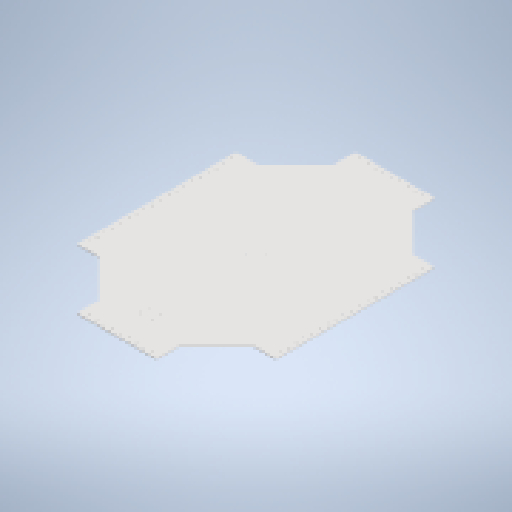
# Autodesk Inventor part: Baseplate V2.1
Saved by Autodesk Inventor 2023 (Build 270158000, 158)
## iProperties
Created: 2023-01-16
Part Number: Baseplate V2.1
Material: Generic
Document SubType Name: Modeling
Designer: Gabriel - T3 CAD
Density: 1 g/cm^3
Appearance: Default
Author: Gabriel - T3 CAD
Autodesk Inventor part; units mm, degrees
ref_plane "YZ Plane" through (0, 0, 0) normal (1, 0, 0) x (0, 1, 0)
ref_plane "XZ Plane" through (0, 0, 0) normal (0, 1, 0) x (-1, 0, 0)
ref_plane "XY Plane" through (0, 0, 0) normal (0, 0, 1) x (1, 0, 0)
sketch "Sketch1" plane through (0, 0, 0) normal (0, 1, 0) x (-1, 0, 0)
  line L0 (0, 0) -> (635, 0)
  line L1 (635, 0) -> (635, 889)
  line L2 (635, 889) -> (0, 889)
  line L3 (0, 889) -> (0, 0)
  line L4 (0, 0) -> (69.85, 0)
  line L5 (69.85, 0) -> (69.85, 190.5)
  line L6 (69.85, 190.5) -> (0, 190.5)
  line L7 (0, 190.5) -> (0, 0)
  line L8 (0, 0) -> (190.5, 0)
  line L9 (190.5, 0) -> (190.5, 69.85)
  line L10 (190.5, 69.85) -> (0, 69.85)
  line L11 (0, 69.85) -> (0, 0)
  line L12 (190.5, 69.85) -> (69.85, 190.5)
  line L13 (317.5, 889) -> (317.5, 0)
  line L14 (0, 444.5) -> (635, 444.5)
  line L15 (565.15, 0) -> (565.15, 190.5)
  line L16 (565.15, 190.5) -> (635, 190.5)
  line L17 (444.5, 0) -> (444.5, 69.85)
  line L18 (444.5, 69.85) -> (635, 69.85)
  line L19 (444.5, 69.85) -> (565.15, 190.5)
  line L20 (69.85, 889) -> (69.85, 698.5)
  line L21 (69.85, 698.5) -> (0, 698.5)
  line L22 (190.5, 889) -> (190.5, 819.15)
  line L23 (190.5, 819.15) -> (0, 819.15)
  line L24 (190.5, 819.15) -> (69.85, 698.5)
  line L25 (565.15, 889) -> (565.15, 698.5)
  line L26 (565.15, 698.5) -> (635, 698.5)
  line L27 (444.5, 889) -> (444.5, 819.15)
  line L28 (444.5, 819.15) -> (635, 819.15)
  line L29 (444.5, 819.15) -> (565.15, 698.5)
  circle A0 centre (622.3, 876.3) radius 2.3813
  circle A1 centre (622.3, 850.9) radius 2.3813
  circle A2 centre (622.3, 825.5) radius 2.3813
  circle A3 centre (622.3, 800.1) radius 2.3813
  circle A4 centre (622.3, 774.7) radius 2.3813
  circle A5 centre (622.3, 749.3) radius 2.3813
  circle A6 centre (622.3, 723.9) radius 2.3813
  circle A7 centre (622.3, 698.5) radius 2.3813
  circle A8 centre (622.3, 673.1) radius 2.3813
  circle A9 centre (622.3, 647.7) radius 2.3813
  circle A10 centre (622.3, 622.3) radius 2.3813
  circle A11 centre (622.3, 596.9) radius 2.3813
  circle A12 centre (622.3, 571.5) radius 2.3813
  circle A13 centre (622.3, 546.1) radius 2.3813
  circle A14 centre (622.3, 520.7) radius 2.3813
  circle A15 centre (622.3, 495.3) radius 2.3813
  circle A16 centre (622.3, 469.9) radius 2.3813
  circle A17 centre (622.3, 444.5) radius 2.3813
  circle A18 centre (622.3, 419.1) radius 2.3813
  circle A19 centre (622.3, 393.7) radius 2.3813
  circle A20 centre (622.3, 368.3) radius 2.3813
  circle A21 centre (622.3, 342.9) radius 2.3813
  circle A22 centre (622.3, 317.5) radius 2.3813
  circle A23 centre (622.3, 292.1) radius 2.3813
  circle A24 centre (622.3, 266.7) radius 2.3813
  circle A25 centre (622.3, 241.3) radius 2.3813
  circle A26 centre (622.3, 215.9) radius 2.3813
  circle A27 centre (622.3, 190.5) radius 2.3813
  circle A28 centre (622.3, 165.1) radius 2.3813
  circle A29 centre (622.3, 139.7) radius 2.3813
  circle A30 centre (622.3, 114.3) radius 2.3813
  circle A31 centre (622.3, 88.9) radius 2.3813
  circle A32 centre (622.3, 63.5) radius 2.3813
  circle A33 centre (622.3, 38.1) radius 2.3813
  circle A34 centre (622.3, 12.7) radius 2.3813
  circle A35 centre (12.7, 876.3) radius 2.3813
  circle A36 centre (12.7, 850.9) radius 2.3813
  circle A37 centre (12.7, 825.5) radius 2.3813
  circle A38 centre (12.7, 800.1) radius 2.3813
  circle A39 centre (12.7, 774.7) radius 2.3813
  circle A40 centre (12.7, 749.3) radius 2.3813
  circle A41 centre (12.7, 723.9) radius 2.3813
  circle A42 centre (12.7, 698.5) radius 2.3813
  circle A43 centre (12.7, 673.1) radius 2.3813
  circle A44 centre (12.7, 647.7) radius 2.3813
  circle A45 centre (12.7, 622.3) radius 2.3813
  circle A46 centre (12.7, 596.9) radius 2.3813
  circle A47 centre (12.7, 571.5) radius 2.3813
  circle A48 centre (12.7, 546.1) radius 2.3813
  circle A49 centre (12.7, 520.7) radius 2.3813
  circle A50 centre (12.7, 495.3) radius 2.3813
  circle A51 centre (12.7, 469.9) radius 2.3813
  circle A52 centre (12.7, 444.5) radius 2.3813
  circle A53 centre (12.7, 419.1) radius 2.3813
  circle A54 centre (12.7, 393.7) radius 2.3813
  circle A55 centre (12.7, 368.3) radius 2.3813
  circle A56 centre (12.7, 342.9) radius 2.3813
  circle A57 centre (12.7, 317.5) radius 2.3813
  circle A58 centre (12.7, 292.1) radius 2.3813
  circle A59 centre (12.7, 266.7) radius 2.3813
  circle A60 centre (12.7, 241.3) radius 2.3813
  circle A61 centre (12.7, 215.9) radius 2.3813
  circle A62 centre (12.7, 190.5) radius 2.3813
  circle A63 centre (12.7, 165.1) radius 2.3813
  circle A64 centre (12.7, 139.7) radius 2.3813
  circle A65 centre (12.7, 114.3) radius 2.3813
  circle A66 centre (12.7, 88.9) radius 2.3813
  circle A67 centre (12.7, 63.5) radius 2.3813
  circle A68 centre (12.7, 38.1) radius 2.3813
  circle A69 centre (12.7, 12.7) radius 2.3813
  circle A70 centre (596.9, 876.3) radius 2.3813
  circle A71 centre (571.5, 876.3) radius 2.3813
  circle A72 centre (546.1, 876.3) radius 2.3813
  circle A73 centre (520.7, 876.3) radius 2.3813
  circle A74 centre (495.3, 876.3) radius 2.3813
  circle A75 centre (469.9, 876.3) radius 2.3813
  circle A76 centre (444.5, 876.3) radius 2.3813
  circle A77 centre (419.1, 876.3) radius 2.3813
  circle A78 centre (393.7, 876.3) radius 2.3813
  circle A79 centre (368.3, 876.3) radius 2.3813
  circle A80 centre (342.9, 876.3) radius 2.3813
  circle A81 centre (317.5, 876.3) radius 2.3813
  circle A82 centre (292.1, 876.3) radius 2.3813
  circle A83 centre (266.7, 876.3) radius 2.3813
  circle A84 centre (241.3, 876.3) radius 2.3813
  circle A85 centre (215.9, 876.3) radius 2.3813
  circle A86 centre (190.5, 876.3) radius 2.3813
  circle A87 centre (165.1, 876.3) radius 2.3813
  circle A88 centre (139.7, 876.3) radius 2.3813
  circle A89 centre (114.3, 876.3) radius 2.3813
  circle A90 centre (88.9, 876.3) radius 2.3813
  circle A91 centre (63.5, 876.3) radius 2.3813
  circle A92 centre (38.1, 876.3) radius 2.3813
  circle A93 centre (12.7, 876.3) radius 2.3813
  circle A94 centre (622.3, 12.7) radius 2.3813
  circle A95 centre (596.9, 12.7) radius 2.3813
  circle A96 centre (571.5, 12.7) radius 2.3813
  circle A97 centre (546.1, 12.7) radius 2.3813
  circle A98 centre (520.7, 12.7) radius 2.3813
  circle A99 centre (495.3, 12.7) radius 2.3813
  circle A100 centre (469.9, 12.7) radius 2.3813
  circle A101 centre (444.5, 12.7) radius 2.3813
  circle A102 centre (419.1, 12.7) radius 2.3813
  circle A103 centre (393.7, 12.7) radius 2.3813
  circle A104 centre (368.3, 12.7) radius 2.3813
  circle A105 centre (342.9, 12.7) radius 2.3813
  circle A106 centre (317.5, 12.7) radius 2.3813
  circle A107 centre (292.1, 12.7) radius 2.3813
  circle A108 centre (266.7, 12.7) radius 2.3813
  circle A109 centre (241.3, 12.7) radius 2.3813
  circle A110 centre (215.9, 12.7) radius 2.3813
  circle A111 centre (190.5, 12.7) radius 2.3813
  circle A112 centre (165.1, 12.7) radius 2.3813
  circle A113 centre (139.7, 12.7) radius 2.3813
  circle A114 centre (114.3, 12.7) radius 2.3813
  circle A115 centre (88.9, 12.7) radius 2.3813
  circle A116 centre (63.5, 12.7) radius 2.3813
  circle A117 centre (38.1, 12.7) radius 2.3813
  circle A118 centre (12.7, 12.7) radius 2.3813
  point P0 (0, 698.5)
  dimension "d0" = 635
  dimension "d1" = 889
  dimension "d2" = 69.85
  dimension "d3" = 190.5
  dimension "d4" = 190.5
  dimension "d5" = 69.85
  dimension "d6" = 317.5
  dimension "d7" = 444.5
  dimension "d8" = 12.7
  dimension "d9" = 12.7
  dimension "d10" = 4.7625
  dimension "d13" = 25.4
  dimension "d16" = 609.6
  dimension "d21" = 25.4
  dimension "d24" = 863.6
  constraints: 119 centre point, 60 end point, 18 symmetric about line, 6 parallel, 5 horizontal, 5 perpendicular, 4 midpoint, 2 vertical, 236 other
  measures "d0" distance of L2.end L1.end
  measures "d1" distance of L1.end L0.end
  measures "d2" distance of L6.end L5.end
  measures "d3" distance of L5.end L4.end
  measures "d4" distance of L10.end L9.end
  measures "d5" distance of L9.end L8.end
  measures "d6" distance between parallel lines of L3 L13
  measures "d7" distance between parallel lines of L2 L14
  measures "d8" distance from line of A0.centre L1
  measures "d9" distance from line of L2 A0.centre
  measures "d10" diameter of A0
  measures "d13" distance of A0.centre A1.centre
  measures "d16" distance of A0.centre A35.centre
  measures "d21" distance of A0.centre A70.centre
  measures "d24" distance of A0.centre A94.centre
extrude "Extrusion1" add sketch "Sketch1" along normal blind 3.175 contours L9 A111 L12 L6 A62 L3 L14 A52 L13 A106 L0 | L13 A106 L14 A17 L1 L16 A27 L19 L17 A101 L0 | L9 A111 | L3 L21 A42 L24 L22 A86 L2 L13 A81 L14 A52 | A62 L6 | A101 L17 | L21 A42 | L13 A81 L2 L27 A76 L29 L26 A7 L1 L14 A17 | A27 L16 | L22 A86 | A7 L26 | L27 A76 picked at (191.8094, 13.1949) picked at (12.7957, 191.288) picked at (443.9736, 12.1059) picked at (13.1509, 697.8467) picked at (622.8941, 191.4063) picked at (191.3482, 876.9206) picked at (622.9275, 697.1304) picked at (442.6593, 876.2043)
sketch "Sketch3" plane through (0, 3.175, 0) normal (0, 1, 0) x (1, 0, 0)
  circle A0 centre (-342.9, -787.4) radius 2.3812
  line L0 (-470.4399, -952.6982) -> (-415.935, -952.6982)
  line L1 (-415.935, -952.6982) -> (-415.935, -907.4708)
  circle A1 centre (-304.8, -787.4) radius 2.3812
  circle A2 centre (-342.9, -762) radius 2.3812
  circle A3 centre (-304.8, -762) radius 2.3812
  line L2 (-444.5, -889) -> (-190.5, -889) projected
  line L3 (-444.5, -819.15) -> (-444.5, -889) projected
  point P0 (0, 0)
  dimension "d42" = 38.1
  dimension "d45" = 25.4
  dimension "d48" = 4.7625
  dimension "d51" = 101.6
  dimension "d52" = 101.6
  constraints: 4 centre point, 4 end point, 1 horizontal, 1 perpendicular, 1 vertical, 6 other
  measures "d42" distance of A0.centre A1.centre
  measures "d45" distance of A0.centre A2.centre
  measures "d48" diameter of A0
  measures "d51" distance from line of L2 A0.centre
  measures "d52" distance from line of L3 A0.centre
extrude "Extrusion3" cut sketch "Sketch3" against normal blind 25.4
sketch "Sketch4" plane through (0, 3.175, 0) normal (0, 1, 0) x (1, 0, 0)
  line L0 (-331.978, -458.978) -> (-303.022, -458.978)
  line L1 (-303.022, -458.978) -> (-303.022, -430.022)
  line L2 (-303.022, -430.022) -> (-331.978, -430.022)
  line L3 (-331.978, -430.022) -> (-331.978, -458.978)
  circle A0 centre (-303.022, -430.022) radius 1.6319
  circle A1 centre (-331.978, -430.022) radius 1.6319
  circle A2 centre (-331.978, -458.978) radius 1.6319
  circle A3 centre (-303.022, -458.978) radius 1.6319
  line L4 (0, -698.5) -> (0, -190.5) projected
  line L5 (-190.5, 0) -> (-444.5, 0) projected
  point P0 (0, 0)
  dimension "d53" = 28.956
  dimension "d54" = 28.956
  dimension "d55" = 3.2639
  dimension "d56" = 3.2639
  dimension "d57" = 3.2639
  dimension "d58" = 3.2639
  dimension "d59" = 303.022
  dimension "d60" = 430.022
  constraints: 8 end point, 4 centre point, 4 coincident, 2 parallel, 1 horizontal, 1 perpendicular
  measures "d53" distance of L1.end L2.end
  measures "d54" distance of L0.end L1.end
  measures "d55" diameter of A3
  measures "d56" diameter of A2
  measures "d57" diameter of A1
  measures "d58" diameter of A0
  measures "d59" distance between parallel lines of L4 L1
  measures "d60" distance between parallel lines of L5 L2
extrude "Extrusion4" cut sketch "Sketch4" against normal blind 25.4 contours L3 A2 L0 | L0 A2 L3 | A3 L1 L0 | L0 L1 A3 | A1 L2 L3 | L3 L2 A1 | A0 L2 L1 | L1 L2 A0
equation "\"d6\" = 0.5 * d0"
equation "\"d7\" = 0.5 * d1"
equation "\"d54\" = d53"
equation "\"d56\" = d55"
equation "\"d57\" = d55"
equation "\"d58\" = d55"
body "Solid1"
